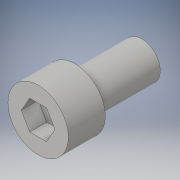
# Autodesk Inventor part: shcs-6-0250
Saved by Autodesk Inventor 2016 (Build 200138000, 138)
## iProperties
Created: 2016-07-01
Part Number: shcs-6-0250
Material: Generic
Document SubType Name: Modeling
Designer: rickab1
Density: 1 g/cm^3
Appearance: Default
Author: rickab1
Autodesk Inventor part; units mm, degrees
ref_plane "YZ Plane" through (0, 0, 0) normal (1, 0, 0) x (0, 1, 0)
ref_plane "XZ Plane" through (0, 0, 0) normal (0, 1, 0) x (-1, 0, 0)
ref_plane "XY Plane" through (0, 0, 0) normal (0, 0, 1) x (1, 0, 0)
sketch "Sketch1" plane through (0, 0, 0) normal (0, 0, 1) x (1, 0, 0)
  circle A0 centre (0, 0) radius 2.8702
  dimension "head_dia" = 5.7404
  constraints: 1 centre point, 1 coincident
  measures "head_dia" diameter of A0
extrude "Extrusion1" add sketch "Sketch1" against normal blind 3.5052
sketch "Sketch2" plane through (0, 0, -3.5052) normal (0, 0, -1) x (-1, 0, 0)
  circle A0 centre (0, 0) radius 1.7526
  dimension "body_dia" = 3.5052
  constraints: 1 centre point, 1 coincident
  measures "body_dia" diameter of A0
extrude "Extrusion2" add sketch "Sketch2" along normal blind 6.35
sketch "Sketch3" plane through (0, 0, 0) normal (0, 0, 1) x (1, 0, 0)
  line L0 (1.604, 0) -> (0.802, -1.3891)
  line L1 (0.802, -1.3891) -> (-0.802, -1.3891)
  line L2 (-0.802, -1.3891) -> (-1.604, 0)
  line L3 (-1.604, 0) -> (-0.802, 1.3891)
  line L4 (-0.802, 1.3891) -> (0.802, 1.3891)
  line L5 (0.802, 1.3891) -> (1.604, 0)
  point P0 (0, 0)
  point P1 (0, 0)
  dimension "allen" = 2.7781
  constraints: 12 end point, 1 coincident, 1 horizontal alignment, 13 other
  measures "allen" distance between parallel lines of L1 L4
extrude "Extrusion3" cut sketch "Sketch3" against normal blind 1.6256
body "Solid1"
